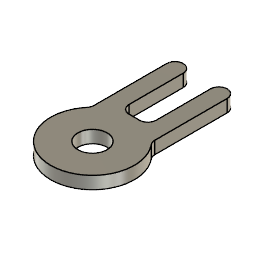
smartie_hopper_servo_arm (Autodesk Fusion 360 design; units mm, degrees)
part number: 2026-05-20-12-12-58-237
Autodesk Fusion 360 part; units mm, degrees
sketch "Smartie Hopper servo arm" plane through (0, 0, 0) normal (0, 0, 1) x (1, 0, 0)
  circle A0 centre (0, 0) radius 10
  circle A1 centre (0, 0) radius 3.5
  line L0 (-3.25, 25) -> (-3.25, 10)
  line L1 (3.25, 25) -> (3.25, 10)
  line L2 (-7.25, 25) -> (-7.25, 6.8875)
  line L3 (7.25, 25) -> (7.25, 6.8875)
  line L4 (-3.25, 10) -> (3.25, 10)
  line L5 (-7.25, 25) -> (-3.25, 25)
  line L6 (3.25, 25) -> (7.25, 25)
  circle A2 centre (-5.25, 25) radius 2
  circle A3 centre (5.25, 25) radius 2
  dimension "d3" = 7
  dimension "d5" = 20
  dimension "d28" = 3.25
  dimension "d29" = 3.25
  dimension "d34" = 4
  dimension "d35" = 4
  dimension "d36" = 15
  dimension "d37" = 15
  dimension "d38" = 4
  dimension "d39" = 4
  constraint coincident A0.centre A1.centre
  constraint concentric A0 A1
  constraint vertical L0
  constraint coincident A0 L2.end
  constraint vertical L2
  constraint coincident A0 L3.end
  constraint parallel L2 L3
  constraint perpendicular L1 L4
  constraint tangent A0 L4
  constraint perpendicular L0 L5
  constraint coincident L1 L6.start
  constraint perpendicular L1 L6
  constraint midpoint L5 A2.centre
  constraint midpoint L6 A3.centre
  constraint horizontal L4
  measures "d3" diameter of A1
  measures "d5" diameter of A0
  measures "d28" horizontal distance of A0.centre L0.end
  measures "d29" horizontal distance of A0.centre L1.end
  measures "d34" diameter of A2
  measures "d35" diameter of A3
  measures "d36" distance of L4 A3.centre
  measures "d37" distance of L4 A2.centre
  measures "d38" distance of L0 L2
  measures "d39" distance of L1 L3
extrude "Extrude1" add sketch "Smartie Hopper servo arm" along normal blind 3
fillet "Fillet4" radius 2 2 edges at (3.25, 10, 1.5) (-3.25, 10, 1.5)
fillet "Fillet3" radius 2 2 edges at (7.25, 6.8875, 1.5) (-7.25, 6.8875, 1.5)
equation "stainless_steel_thickness = 3 mm" comment "The thickness of the 316 stainless steel sheets to laser cut."
equation "arm_thickness = 4 mm"
equation "d10 = stainless_steel_thickness"
equation "groove_diameter = 6.5 mm"
equation "groove_length = 17 mm"
equation "d28 = groove_diameter / 2"
equation "d29 = groove_diameter / 2"
equation "d34 = arm_thickness"
equation "d35 = arm_thickness"
equation "d36 = groove_length - ( arm_thickness / 2 )"
equation "d37 = groove_length - ( arm_thickness / 2 )"
equation "d38 = arm_thickness"
equation "d39 = arm_thickness"
named bodies: "Smartie Hopper servo arm"
